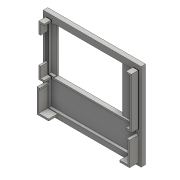
# Autodesk Inventor part: ARDUINO_DUE_CASE_TOP_NEU
Saved by Autodesk Inventor 2016 (Build 200138000, 138)
## iProperties
Created: 2015-06-07
Part Number: ARDUINO_DUE_CASE_TOP_NEU
Material: Generic
Document SubType Name: Modeling
Designer: Admin
Density: 1 g/cm^3
Appearance: Default
Author: Admin
Autodesk Inventor part; units mm, degrees
ref_plane "YZ Plane" through (0, 0, 0) normal (1, 0, 0) x (0, 1, 0)
ref_plane "XZ Plane" through (0, 0, 0) normal (0, 1, 0) x (-1, 0, 0)
ref_plane "XY Plane" through (0, 0, 0) normal (0, 0, 1) x (1, 0, 0)
sketch "Skizze1" plane through (0, 0, 0) normal (0, 1, 0) x (-1, 0, 0)
  line L0 (0, 0) -> (-110, 0)
  line L1 (-110, 0) -> (-110, 98)
  line L2 (-110, 98) -> (0, 98)
  line L3 (0, 98) -> (0, 0)
  dimension "d0" = 110
  dimension "d1" = 98
  constraints: 8 end point, 2 parallel, 1 horizontal, 1 perpendicular
  measures "d0" distance of L1.end L2.end
  measures "d1" distance of L0.end L1.end
extrude "Extrusion1" add sketch "Skizze1" along normal blind 5
sketch "Skizze2" plane through (0, 0, 0) normal (0, -1, 0) x (1, 0, 0)
  line L0 (107, 93) -> (105, 93)
  line L1 (105, 93) -> (105, 36)
  line L2 (105, 36) -> (107, 36)
  line L3 (107, 36) -> (107, 93)
  line L4 (3, 93) -> (5, 93)
  line L5 (5, 93) -> (5, 36)
  line L6 (5, 36) -> (3, 36)
  line L7 (3, 36) -> (3, 93)
  line L8 (5, 36) -> (9, 36)
  line L9 (9, 36) -> (9, 38)
  line L10 (9, 38) -> (5, 38)
  line L11 (5, 38) -> (5, 36)
  line L12 (5, 93) -> (9, 93)
  line L13 (9, 93) -> (9, 91)
  line L14 (9, 91) -> (5, 91)
  line L15 (5, 91) -> (5, 93)
  line L16 (105, 93) -> (101, 93)
  line L17 (101, 93) -> (101, 91)
  line L18 (101, 91) -> (105, 91)
  line L19 (105, 91) -> (105, 93)
  line L20 (105, 36) -> (101, 36)
  line L21 (101, 36) -> (101, 38)
  line L22 (101, 38) -> (105, 38)
  line L23 (105, 38) -> (105, 36)
  constraints: 48 end point, 12 parallel, 6 horizontal, 6 perpendicular, 6 point on line
extrude "Extrusion2" add sketch "Skizze2" along normal blind 8 contours L3 L2 L1 L0
extrude "Extrusion3" add sketch "Skizze2" along normal blind 8 contours L20 L21 L22 L1
extrude "Extrusion4" add sketch "Skizze2" along normal blind 8 contours L1 L18 L17 L16
extrude "Extrusion5" add sketch "Skizze2" along normal blind 8 contours L5 L10 L9 L8
extrude "Extrusion6" add sketch "Skizze2" along normal blind 8 contours L4 L5 L6 L7
extrude "Extrusion7" add sketch "Skizze2" along normal blind 8 contours L12 L13 L14 L5
sketch "Skizze3" plane through (0, -8, 0) normal (0, -1, 0) x (1, 0, 0)
  line L0 (5, 38) -> (5, 91) projected
  line L1 (3, 93) -> (3, 36) projected
  line L2 (3, 80) -> (5, 80)
  line L3 (5, 80) -> (5, 50)
  line L4 (5, 50) -> (3, 50)
  line L5 (3, 50) -> (3, 80)
  point P0 (0, 0)
  constraints: 8 end point, 2 parallel, 2 point on line, 1 horizontal, 1 perpendicular
extrude "Extrusion8" cut sketch "Skizze3" against normal blind 8
sketch "Skizze4" plane through (0, 5, 0) normal (0, 1, 0) x (1, 0, 0)
  line L0 (12.0049, -91) -> (87.0387, -91)
  line L1 (87.0387, -91) -> (87.0387, -37.9492)
  line L2 (87.0387, -37.9492) -> (12.0049, -37.9492)
  line L3 (12.0049, -37.9492) -> (12.0049, -91)
  constraints: 8 end point, 2 parallel, 1 horizontal, 1 perpendicular
extrude "Extrusion9" cut sketch "Skizze4" against normal blind 8
sketch "Skizze5" plane through (0, 0, 0) normal (0, -1, 0) x (1, 0, 0)
  line L0 (3, 3) -> (107, 3)
  line L1 (107, 3) -> (107, 30)
  line L2 (107, 30) -> (3, 30)
  line L3 (3, 30) -> (3, 3)
  constraints: 8 end point, 2 parallel, 1 horizontal, 1 perpendicular
extrude "Extrusion10" add sketch "Skizze5" along normal blind 10
sketch "Skizze6" plane through (0, -10, 0) normal (0, -1, 0) x (1, 0, 0)
  line L0 (5, 5) -> (105, 5)
  line L1 (105, 5) -> (105, 28)
  line L2 (105, 28) -> (5, 28)
  line L3 (5, 28) -> (5, 5)
  point P0 (0, 0)
  constraints: 8 end point, 2 parallel, 1 horizontal, 1 perpendicular
extrude "Extrusion11" cut sketch "Skizze6" against normal blind 10
sketch "Skizze7" plane through (0, -10, 0) normal (0, -1, 0) x (1, 0, 0)
  line L0 (107, 30) -> (3, 30) projected
  line L1 (5, 28) -> (105, 28) projected
  line L2 (14, 30) -> (98, 30)
  line L3 (98, 30) -> (98, 28)
  line L4 (98, 28) -> (14, 28)
  line L5 (14, 28) -> (14, 30)
  point P0 (0, 0)
  constraints: 8 end point, 2 parallel, 2 point on line, 1 horizontal, 1 perpendicular
extrude "Extrusion12" cut sketch "Skizze7" against normal blind 10
sketch "Skizze8" plane through (0, -10, 0) normal (0, -1, 0) x (1, 0, 0)
  line L0 (105, 5) -> (5, 5) projected
  line L1 (107, 3) -> (3, 3) projected
  line L2 (16, 5) -> (96, 5)
  line L3 (96, 5) -> (96, 3)
  line L4 (96, 3) -> (16, 3)
  line L5 (16, 3) -> (16, 5)
  point P0 (0, 0)
  constraints: 8 end point, 2 parallel, 2 point on line, 1 horizontal, 1 perpendicular
extrude "Extrusion13" cut sketch "Skizze8" against normal blind 10
sketch "Skizze14" plane through (0, 0, 0) normal (0, -1, 0) x (1, 0, 0)
  line L0 (87.0387, 37.9492) -> (98, 37.9492)
  line L1 (98, 37.9492) -> (98, 91)
  line L2 (98, 91) -> (87.0387, 91)
  line L3 (87.0387, 91) -> (87.0387, 37.9492)
  constraints: 8 end point, 2 parallel, 1 horizontal, 1 perpendicular
extrude "Extrusion20" cut sketch "Skizze14" against normal blind 2
sketch "Skizze15" plane through (0, 0, 0) normal (0, -1, 0) x (1, 0, 0)
  line L0 (104, 6) -> (6, 6)
  line L1 (6, 6) -> (6, 27)
  line L2 (6, 27) -> (104, 27)
  line L3 (104, 27) -> (104, 6)
  constraints: 8 end point, 2 parallel, 1 horizontal, 1 perpendicular
extrude "Extrusion21" cut sketch "Skizze15" against normal blind 3
sketch "Skizze16" plane through (0, -10, 0) normal (0, -1, 0) x (1, 0, 0)
  line L0 (104, 28) -> (6, 28)
  line L1 (6, 28) -> (6, 30)
  line L2 (6, 30) -> (104, 30)
  line L3 (104, 30) -> (104, 28)
  point P0 (0, 0)
  constraints: 8 end point, 2 parallel, 1 horizontal, 1 perpendicular
extrude "Extrusion22" cut sketch "Skizze16" against normal blind 10
sketch "Skizze17" plane through (0, 0, 0) normal (0, -1, 0) x (1, 0, 0)
  line L0 (9, 36) -> (3, 36) projected
  line L1 (104, 27) -> (6, 27)
  line L2 (6, 27) -> (6, 36)
  line L3 (6, 36) -> (104, 36)
  line L4 (104, 36) -> (104, 27)
  constraints: 8 end point, 2 parallel, 1 horizontal, 1 midpoint, 1 perpendicular
extrude "Extrusion23" cut sketch "Skizze17" against normal blind 3
sketch "Skizze18" plane through (0, 0, 0) normal (0, -1, 0) x (1, 0, 0)
  line L0 (12.0049, 91) -> (12.0049, 37.9492) projected
  line L1 (12.0049, 39) -> (6, 39)
  line L2 (6, 39) -> (6, 90)
  line L3 (6, 90) -> (12.0049, 90)
  line L4 (12.0049, 90) -> (12.0049, 39)
  constraints: 8 end point, 2 parallel, 1 horizontal, 1 perpendicular, 1 point on line
extrude "Extrusion24" cut sketch "Skizze18" against normal blind 3
